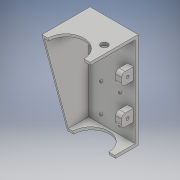
# Autodesk Inventor part: Center_bar_panel
Saved by Autodesk Inventor 2019 (Build 230136000, 136)
## iProperties
Created: 2019-11-07
Part Number: Center_bar_panel
Material: Generic
Document SubType Name: Modeling
Designer: steve
Density: 1 g/cm^3
Appearance: Default
Author: steve
Autodesk Inventor part; units mm, degrees
ref_plane "YZ Plane" through (0, 0, 0) normal (1, 0, 0) x (0, 1, 0)
ref_plane "XY Plane" through (0, 0, 0) normal (0, 0, 1) x (1, 0, 0)
sketch "Sketch1" plane through (0, 0, 0) normal (0, 1, 0) x (-1, 0, 0)
  arc A0 (-60, 0) -> (60, 0) centre (0, 0) ccw
  line L0 (80, 0) -> (80, -75)
  line L1 (80, -75) -> (-80, -75)
  line L2 (-80, -75) -> (-80, 0)
  line L3 (-80, 0) -> (-60, 0)
  line L4 (60, 0) -> (80, 0)
  line L5 (112, 0) -> (-112, 0) projected
  dimension "d1" = 20
  dimension "archRad" = 60
  dimension "d3" = 75
  constraints: 10 end point, 3 perpendicular, 2 collinear, 2 equal length, 2 point on circle, 1 centre point, 1 coincident, 1 vertical
  measures "d1" distance of L4.start L0.start
  measures "archRad" radius of A0
  measures "d3" distance from line of A0.centre L1
ref_plane "Work Plane1" through (0, 10, 0) normal (0, 1, 0) x (-1, 0, 0)
sketch "Sketch2" plane through (0, 10, 0) normal (0, 1, 0) x (-1, 0, 0)
  line L0 (80, -75) -> (-80, -75) projected
  line L1 (80, 0) -> (80, -75) projected
  line L2 (-80, -75) -> (-80, 0) projected
  line L3 (80, 0) -> (80, 2.67)
  line L4 (-80, 2.67) -> (-80, 0)
  arc A0 (-60, 2.67) -> (60, 2.67) centre (0, 2.67) ccw
  line L5 (80, 2.67) -> (60, 2.67)
  line L6 (-60, 2.67) -> (-80, 2.67)
  line L7 (60, 2.67) -> (-60, 2.67) construction
  point P0 (0, 0)
  dimension "d5" = 60
  dimension "d6" = 2.67
  constraints: 10 end point, 2 collinear, 2 horizontal, 2 point on circle, 2 vertical, 1 centre point, 1 coincident, 1 midpoint
  measures "d5" radius of A0
  measures "d6" distance from line of L5 L1.start
loft "Loft1" add profiles "Sketch1", "Sketch2" contours A0 L4 L0 L1 L2 L3 / all
sketch "Sketch3" plane through (0, 10, 2.67) normal (0, 1, 0) x (1, 0, 0)
  line L0 (80, 77.67) -> (80, 2.67) projected
  line L1 (-80, 77.67) -> (80, 77.67)
  line L2 (80, 77.67) -> (80, 67.67)
  line L3 (80, 67.67) -> (-80, 67.67)
  line L4 (-80, 67.67) -> (-80, 77.67)
  point P0 (0, 2.67)
  dimension "d12" = 10
  constraints: 8 end point, 2 parallel, 1 horizontal, 1 perpendicular, 1 point on line
  measures "d12" distance between parallel lines of L1 L3
extrude "Extrusion1" add sketch "Sketch3" along normal blind 300
sketch "Sketch4" plane through (-80, 10, -65) normal (0, 0, 1) x (1, 0, 0)
  line L0 (111.5, 124.8462) -> (48.5, 124.8462) construction
  line L1 (48.5, 124.8462) -> (48.5, 30) construction
  line L2 (48.5, 30) -> (111.5, 30) construction
  line L3 (111.5, 30) -> (111.5, 124.8462) construction
  line L4 (111.5, 124.8462) -> (48.5, 30) construction
  line L5 (48.5, 124.8462) -> (111.5, 30) construction
  line L6 (140, -10) -> (20, -10) construction
  line L7 (160, 0) -> (160, 300) construction
  line L8 (0, 0) -> (0, 300) construction
  circle A0 centre (48.5, 124.8462) radius 4.5
  circle A1 centre (111.5, 124.8462) radius 4.5
  circle A2 centre (111.5, 30) radius 4.5
  circle A3 centre (48.5, 30) radius 4.5
  circle A4 centre (48.5, 124.8462) radius 1.5
  circle A5 centre (111.5, 124.8462) radius 1.5
  circle A6 centre (111.5, 30) radius 1.5
  circle A7 centre (48.5, 30) radius 1.5
  point P0 (80, -10)
  point P1 (80, 77.4231)
  dimension "d15" = 63
  dimension "d16" = 94.8461
  dimension "d17" = 40
  dimension "d18" = 160
  dimension "d19" = 80
  dimension "d20" = 3
  dimension "d21" = 3
  constraints: 12 end point, 8 centre point, 7 coincident, 6 equal radius, 2 midpoint, 2 parallel, 1 concentric, 1 horizontal, 1 perpendicular
  measures "d15" distance of L0.start L0.end
  measures "d16" distance of L2.end L0.start
  measures "d17" distance between parallel lines of L6 L2
  measures "d18" distance between parallel lines of L7 L8
  measures "d19" distance from line of L8 point (80, 77.423)
  measures "d20" radial gap between concentric circles of A4 A0
  measures "d21" diameter of A4
extrude "Extrusion2" add sketch "Sketch4" along normal blind 4
sketch "Sketch5" plane through (80, 0, -75) normal (0, 0, -1) x (-1, 0, 0)
  circle A0 centre (48.5, 40) radius 4.5 projected
  line L0 (111.5, 134.8462) -> (48.5, 134.8462)
  line L1 (48.5, 134.8462) -> (48.5, 40)
  line L2 (48.5, 40) -> (111.5, 40)
  line L3 (111.5, 40) -> (111.5, 134.8462)
  line L4 (111.5, 134.8462) -> (48.5, 40) construction
  line L5 (48.5, 134.8462) -> (111.5, 40) construction
  circle A1 centre (111.5, 40) radius 4.5 projected
  circle A2 centre (111.5, 134.8462) radius 4.5 projected
  line L6 (113.5, 38) -> (46.5, 38)
  line L7 (46.5, 38) -> (46.5, 136.8462)
  line L8 (46.5, 136.8462) -> (113.5, 136.8462)
  line L9 (113.5, 136.8462) -> (113.5, 38)
  point P0 (80, 0)
  point P1 (80, 87.4231)
  dimension "d24" = 2
  constraints: 20 end point, 4 parallel, 2 midpoint, 2 perpendicular, 1 coincident, 1 horizontal, 3 other
  measures "d24" distance between parallel lines of L7 L1
extrude "Extrusion3" cut sketch "Sketch5" against normal blind 1 contours L2 A1 L6 A0 | A0 L6 L7 L1 L2 | A0 L7 L8 A2 L0 L1 | L2 L3 A1 L9 L6 | L3 A2 L9 A1 | A2 L8 L9 L3 L0
sketch "Sketch6" plane through (0, 310, 2.67) normal (0, 1, 0) x (1, 0, 0)
  line L0 (80, 77.67) -> (-80, 77.67) projected
  line L1 (-80, 77.67) -> (-80, -80.1)
  line L2 (80, 67.67) -> (80, 77.67) projected
  line L3 (80, 77.67) -> (80, -80.1)
  arc A0 (60, -80.1) -> (-60, -80.1) centre (0, -80.1) ccw
  line L4 (-80, -80.1) -> (-60, -80.1)
  line L5 (60, -80.1) -> (80, -80.1)
  line L6 (-60, 0) -> (-80, 0) projected
  line L7 (80, 0) -> (60, 0) projected
  point P0 (0, 2.67)
  dimension "d27" = 60
  dimension "d28" = 80.1
  constraints: 8 end point, 2 collinear, 2 equal length, 2 point on circle, 2 vertical, 1 centre point, 1 horizontal
  measures "d27" radius of A0
  measures "d28" distance between parallel lines of L7 L5
ref_plane "Work Plane3" through (0, 320, 2.67) normal (0, 1, 0) x (1, 0, 0)
sketch "Sketch7" plane through (0, 320, 2.67) normal (0, 1, 0) x (1, 0, 0)
  line L0 (80, 77.67) -> (-80, 77.67) projected
  line L1 (-80, 77.67) -> (-80, -80.1) projected
  line L2 (80, 77.67) -> (80, -80.1) projected
  line L3 (-80, -80.1) -> (-80, -82.77)
  arc A0 (60, -82.77) -> (-60, -82.77) centre (0, -82.77) ccw
  line L4 (-80, -82.77) -> (-60, -82.77)
  line L5 (60, -82.77) -> (80, -82.77)
  line L6 (80, -82.77) -> (80, -80.1)
  line L7 (-60, -82.77) -> (60, -82.77) construction
  point P0 (0, 2.67)
  point P1 (50, -9)
  dimension "d37" = 2.67
  dimension "d38" = 60
  constraints: 10 end point, 2 equal length, 2 point on circle, 1 centre point, 1 coincident, 1 collinear, 1 horizontal, 1 midpoint, 1 perpendicular, 1 point on line, 1 vertical
  measures "d37" distance of L1.end L3.end
  measures "d38" radius of A0
loft "Loft2" add profiles "Sketch6", "Sketch7"
sketch "Sketch8" plane through (0, 320, 85.44) normal (0, 1, 0) x (1, 0, 0)
  circle A0 centre (54, 74) radius 11.6619
  point P0 (0, 85.44)
  constraints: 1 centre point
extrude "Extrusion4" cut sketch "Sketch8" against normal up to next
sketch "Sketch9" plane through (-80, 0, -75) normal (-1, 0, 0) x (0, 0, 1)
  line L0 (77.67, 10) -> (10, 10) projected
  line L1 (10, 310) -> (157.77, 310) projected
  line L2 (10, 10) -> (10, 310) projected
  line L3 (157.77, 310) -> (160.44, 320) projected
  line L4 (77.67, 10) -> (157.77, 310)
  point P0 (75, 0)
  constraints: 2 end point, 1 collinear
extrude "Extrusion5" add sketch "Sketch9" against normal blind 5
sketch "Sketch10" plane through (80, 10, -65) normal (0, 0, 1) x (1, 0, 0)
  line L0 (-25, 220) -> (-5, 220)
  line L1 (-5, 220) -> (-5, 180)
  line L2 (-5, 180) -> (-25, 180)
  line L3 (-25, 180) -> (-25, 220)
  line L4 (-25, 100) -> (-5, 100)
  line L5 (-5, 100) -> (-5, 60)
  line L6 (-5, 60) -> (-25, 60)
  line L7 (-25, 60) -> (-25, 100)
  line L8 (0, 0) -> (0, 300) projected
  line L9 (0, 0) -> (-20, 0) projected
  point P0 (-80, -10)
  dimension "d47" = 80
  dimension "d48" = 20
  dimension "d49" = 40
  dimension "d50" = 5
  dimension "d51" = 60
  constraints: 16 end point, 4 parallel, 2 horizontal, 2 perpendicular, 2 point on line, 1 collinear
  measures "d47" distance between parallel lines of L4 L2
  measures "d48" distance of L0.start L0.end
  measures "d49" distance of L0.end L1.end
  measures "d50" distance between parallel lines of L8 L1
  measures "d51" distance between parallel lines of L9 L6
extrude "Extrusion6" add sketch "Sketch10" along normal blind 40
sketch "Sketch11" plane through (75, 190, -65) normal (1, 0, 0) x (0, 0, -1)
  circle A0 centre (-20, 20) radius 5
  circle A1 centre (-20, -100) radius 5
  line L0 (0, -120) -> (-40, -120) projected
  line L1 (0, -80) -> (-40, -80) projected
  line L2 (0, -180) -> (0, 120) projected
  line L3 (-40, -120) -> (-40, -80) projected
  line L4 (0, 0) -> (-40, 0) projected
  line L5 (0, 40) -> (-40, 40) projected
  point P0 (-65, -190)
  dimension "d54" = 40
  dimension "d55" = 40
  dimension "d56" = 20
  dimension "d57" = 20
  dimension "d58" = 0
  dimension "d59" = 40
  dimension "d60" = 20
  dimension "d61" = 10
  constraints: 2 centre point, 1 equal radius
  measures "d54" distance between parallel lines of L0 L1
  measures "d55" distance between parallel lines of L2 L3
  measures "d56" distance from line of L3 A1.centre
  measures "d57" distance from line of A1.centre L1
  measures "d58" horizontal distance of A1.centre A0.centre
  measures "d59" distance between parallel lines of L4 L5
  measures "d60" distance from line of L5 A0.centre
  measures "d61" diameter of A1
extrude "Extrusion7" cut sketch "Sketch11" against normal up to next contours A0 | A1
fillet "Fillet1" radius 11.75 4 edges at (65, 190, -25) (65, 230, -25) (65, 110, -25) (65, 70, -25)
equation "\"d5\" = archRad"
equation "\"d19\" = 0.5 * d18"
equation "\"d27\" = archRad"
equation "\"d38\" = archRad"
equation "\"d56\" = 0.5 * d55"
equation "\"d57\" = 0.5 * d54"
equation "\"d60\" = 0.5 * d59"
equation "\"slope\" = 0.267"
body "Solid1"
